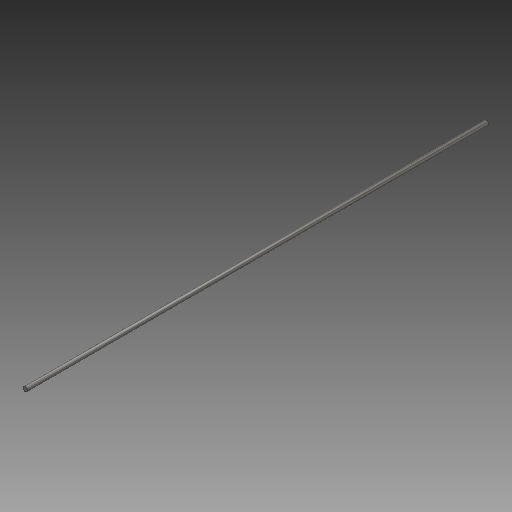
# Autodesk Inventor part: Quick Shaft 12mm x 500mm
Saved by Autodesk Inventor 2017 SP1 (Build 210196100, 196)
## iProperties
Created: 2017-08-08
Part Number: Quick Shaft 12mm x 500mm
Material: Steel, Carbon
Document SubType Name: Modeling
Designer: Zach
Density: 7.85 g/cm^3
Appearance: Semi-Polished
Mass: 616.538 g
Surface Area: 315.73 cm^2
Volume: 78.5398 cm^3
Author: Zach
Autodesk Inventor part; units mm, degrees
ref_plane "YZ Plane" through (0, 0, 0) normal (1, 0, 0) x (0, 1, 0)
ref_plane "XZ Plane" through (0, 0, 0) normal (0, 1, 0) x (-1, 0, 0)
ref_plane "XY Plane" through (0, 0, 0) normal (0, 0, 1) x (1, 0, 0)
sketch "Sketch1" plane through (0, 0, 0) normal (0, 0, 1) x (1, 0, 0)
  circle A0 centre (0, 0) radius 5
  dimension "d0" = 10
  constraints: 1 centre point, 1 coincident
  measures "d0" diameter of A0
extrude "Extrusion1" add sketch "Sketch1" along normal blind 1000
body "Solid1"
